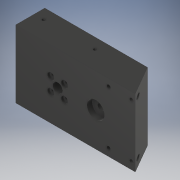
# Autodesk Inventor part: BA03
Saved by Autodesk Inventor 2017 (Build 210142000, 142)
## iProperties
Created: 2018-10-18
Part Number: BA03
Material: ABS Plastic
Document SubType Name: Modeling
Designer: Administrator
Density: 1.06 g/cm^3
Appearance: Smooth - Black
Author: Administrator
Autodesk Inventor part; units mm, degrees
ref_plane "YZ Plane" through (0, 0, 0) normal (1, 0, 0) x (0, 1, 0)
ref_plane "XZ Plane" through (0, 0, 0) normal (0, 1, 0) x (-1, 0, 0)
ref_plane "XY Plane" through (0, 0, 0) normal (0, 0, 1) x (1, 0, 0)
sketch "Sketch1" plane through (0, 0, 0) normal (0, 0, 1) x (1, 0, 0)
  line L0 (0, 0) -> (110, 0)
  line L1 (110, 0) -> (110, 75)
  line L2 (110, 75) -> (0, 75)
  line L3 (0, 75) -> (0, 0)
  circle A0 centre (80, 30.55) radius 4.5
  circle A1 centre (30, 30.55) radius 4
  line L4 (30, 30.55) -> (80, 30.55) construction
  dimension "d0" = 110
  dimension "d1" = 75
  dimension "d2" = 9
  dimension "d3" = 8
  dimension "d4" = 50
  dimension "d5" = 30
  dimension "d80" = 44.45
  constraints: 10 end point, 2 centre point, 2 horizontal, 2 parallel, 1 perpendicular
  measures "d0" distance of L2.end L1.end
  measures "d1" distance of L1.end L0.end
  measures "d2" diameter of A0
  measures "d3" diameter of A1
  measures "d4" distance of L4.start L4.end
  measures "d5" distance from line of L1 L4.end
  measures "d80" distance between parallel lines of L2 L4
extrude "Extrusion1" add sketch "Sketch1" along normal blind 10
sketch "Sketch2" plane through (0, 75, 0) normal (0, 1, 0) x (1, 0, 0)
  line L0 (110, -10) -> (0, -10) projected
  line L1 (0, -10) -> (110, -10)
  line L2 (110, -10) -> (110, 28.1)
  line L3 (110, 28.1) -> (0, 28.1)
  line L4 (0, 28.1) -> (0, -10)
  point P0 (0, 0)
  dimension "d8" = 38.1
  constraints: 8 end point, 2 parallel, 1 horizontal, 1 perpendicular
  measures "d8" distance of L3.end L0.end
extrude "Extrusion2" add sketch "Sketch2" against normal blind 10
sketch "Sketch3" plane through (110, 0, 10) normal (1, 0, 0) x (0, 0, -1)
  line L0 (38.1, 65) -> (10, 65) projected
  line L1 (10, 0) -> (10, 65) projected
  line L2 (10, 0) -> (38.1, 65)
  constraints: 2 end point
extrude "Extrusion3" add sketch "Sketch3" against normal blind 10
sketch "Sketch4" plane through (0, 0, 10) normal (-1, 0, 0) x (0, 0, 1)
  line L0 (-10, 65) -> (-10, 0) projected
  line L1 (-38.1, 65) -> (-10, 65) projected
  line L2 (-38.1, 65) -> (-10, 0) projected
  point P0 (-10, 0)
extrude "Extrusion4" add sketch "Sketch4" against normal blind 10
sketch "Sketch6" plane through (0, 65, 0) normal (0, -1, 0) x (1, 0, 0)
  line L0 (110, -28.1) -> (110, 10) projected
  line L1 (110, 0) -> (135, 0)
  line L2 (135, 0) -> (135, -28.1)
  line L3 (135, -28.1) -> (110, -28.1)
  line L4 (110, -28.1) -> (110, 0)
  line L5 (0, 0) -> (-25, 0)
  line L6 (-25, 0) -> (-25, -28.1)
  line L7 (-25, -28.1) -> (0, -28.1)
  line L8 (0, -28.1) -> (0, 0)
  line L9 (10, -28.1) -> (100, -28.1) projected
  circle A0 centre (122.5, -14.05) radius 2
  circle A1 centre (-12.5, -14.05) radius 2
  point P0 (135, -14.05)
  point P1 (-25, -14.05)
  point P2 (-12.5, -28.1)
  point P3 (122.5, -28.1)
  dimension "d17" = 25
  dimension "d18" = 25
  dimension "d19" = 4
  dimension "d20" = 4
  constraints: 16 end point, 4 horizontal alignment, 4 midpoint, 4 parallel, 2 centre point, 2 horizontal, 2 perpendicular, 2 vertical alignment, 1 coincident, 1 point on line
  measures "d17" distance of L6.end L7.end
  measures "d18" distance of L2.end L3.end
  measures "d19" diameter of A0
  measures "d20" diameter of A1
extrude "Extrusion5" add sketch "Sketch6" against normal blind 10
sketch "Sketch7" plane through (0, 65, 0) normal (0, -1, 0) x (1, 0, 0)
  line L0 (110, 0) -> (135, 0) projected
  line L1 (110, 0) -> (135, 0)
  line L2 (135, 0) -> (135, 10)
  line L3 (135, 10) -> (110, 10)
  line L4 (110, 10) -> (110, 0)
  line L5 (0, 0) -> (10, 0) projected
  line L6 (0, 0) -> (-25, 0)
  line L7 (-25, 0) -> (-25, 10)
  line L8 (-25, 10) -> (0, 10)
  line L9 (0, 10) -> (0, 0)
  point P0 (0, 10)
  point P1 (-25, 0)
  constraints: 16 end point, 4 parallel, 2 horizontal, 2 horizontal alignment, 2 perpendicular, 2 vertical alignment
extrude "Extrusion6" add sketch "Sketch7" against normal blind 10
sketch "Sketch8" plane through (0, 65, 0) normal (0, -1, 0) x (1, 0, 0)
  circle A0 centre (122.5, -14.05) radius 2 projected
  line L0 (10, -28.1) -> (100, -28.1) projected
  circle A1 centre (55, -14.05) radius 2
  point P0 (0, 0)
  point P1 (55, -28.1)
  dimension "d25" = 4
  constraints: 1 centre point, 1 horizontal alignment, 1 midpoint, 1 vertical alignment
  measures "d25" diameter of A1
extrude "Extrusion7" cut sketch "Sketch8" against normal through all contours A1
sketch "Sketch11" plane through (0, 0, 10) normal (0, 0, 1) x (1, 0, 0)
  line L0 (30, 23.55) -> (45.5, 23.55) construction
  circle A0 centre (30, 30.55) radius 4 construction
  circle A1 centre (45.5, 23.55) radius 1.5
  line L1 (30, 23.55) -> (37.75, 36.9734) construction
  circle A2 centre (37.75, 36.9734) radius 1.5
  line L2 (30, 23.55) -> (22.25, 36.9734) construction
  circle A3 centre (22.25, 36.9734) radius 1.5
  line L3 (30, 23.55) -> (14.5, 23.55) construction
  circle A4 centre (14.5, 23.55) radius 1.5
  line L4 (30, 23.55) -> (22.25, 10.1266) construction
  circle A5 centre (22.25, 10.1266) radius 1.5
  line L5 (30, 23.55) -> (37.75, 10.1266) construction
  circle A6 centre (37.75, 10.1266) radius 1.5
  point P0 (0, 0)
  dimension "d31" = 15.5
  dimension "d32" = 7
  dimension "d33" = 3
  dimension "d36" = 360
  constraints: 12 end point, 8 coincident, 6 centre point, 1 horizontal, 1 vertical alignment, 29 other
  measures "d31" distance of L0.start L0.end
  measures "d32" distance of L0.start A0.centre
  measures "d33" diameter of A1
extrude "Extrusion9" cut sketch "Sketch11" against normal through all
sketch "Sketch12" plane through (0, 0, 0) normal (0, 0, -1) x (-1, 0, 0)
  circle A0 centre (-30, 30.55) radius 4 projected
  circle A1 centre (-30, 30.55) radius 6.5
  point P0 (0, 0)
  dimension "d40" = 13
  constraints: 1 centre point, 1 coincident
  measures "d40" diameter of A1
extrude "Extrusion10" cut sketch "Sketch12" against normal through all
sketch "Sketch13" plane through (0, 0, 10) normal (0, 0, 1) x (1, 0, 0)
  circle A0 centre (45.5, 23.55) radius 1.5 projected
  circle A1 centre (14.5, 23.55) radius 1.5 projected
  circle A2 centre (22.25, 36.9734) radius 1.5 projected
  circle A3 centre (37.75, 36.9734) radius 1.5 projected
  circle A4 centre (37.75, 10.1266) radius 1.5 projected
  circle A5 centre (22.25, 10.1266) radius 1.5 projected
  circle A6 centre (14.5, 23.55) radius 4
  circle A7 centre (22.25, 36.9734) radius 4
  circle A8 centre (37.75, 36.9734) radius 4
  circle A9 centre (45.5, 23.55) radius 4
  circle A10 centre (37.75, 10.1266) radius 4
  circle A11 centre (22.25, 10.1266) radius 4
  point P0 (0, 0)
  dimension "d43" = 8
  dimension "d44" = 8
  dimension "d45" = 8
  dimension "d46" = 8
  dimension "d47" = 8
  dimension "d48" = 8
  constraints: 6 centre point, 6 coincident
  measures "d43" diameter of A6
  measures "d44" diameter of A7
  measures "d45" diameter of A8
  measures "d46" diameter of A9
  measures "d47" diameter of A10
  measures "d48" diameter of A11
extrude "Extrusion11" cut sketch "Sketch13" against normal blind 3 contours A0 | A1 | A2 | A3 | A4 | A5 | A6 | A7 | A8 | A9 | A10 | A11
sketch "Sketch15" plane through (0, 0, 10) normal (0, 0, 1) x (1, 0, 0)
  line L0 (135, 75) -> (-25, 75) projected
  line L1 (110, 75) -> (0, 75)
  line L2 (0, 75) -> (0, -13.9)
  line L3 (0, -13.9) -> (110, -13.9)
  line L4 (110, -13.9) -> (110, 75)
  line L5 (100, 0) -> (110, 0) projected
  line L6 (110, 0) -> (0, 0)
  line L7 (0, 0) -> (0, -13.9)
  line L8 (0, -13.9) -> (110, -13.9)
  line L9 (110, -13.9) -> (110, 0)
  dimension "d54" = 88.9
  constraints: 16 end point, 4 parallel, 2 horizontal, 2 perpendicular, 2 vertical alignment, 1 point on line
  measures "d54" distance between parallel lines of L0 L3
extrude "Extrusion13" add sketch "Sketch15" against normal blind 10 contours L4 L3 L2 L6 L5
sketch "Sketch16" plane through (0, -13.9, 10) normal (0, -1, 0) x (1, 0, 0)
  line L0 (0, 0) -> (0, -38.1) projected
  line L1 (10, -10) -> (10, -38.1) projected
  line L2 (0, 0) -> (10, 0)
  line L3 (10, 0) -> (10, -38.1)
  line L4 (10, -38.1) -> (0, -38.1)
  line L5 (0, -38.1) -> (0, 0)
  line L6 (135, 0) -> (110, 0) projected
  line L7 (100, -38.1) -> (100, -10) projected
  line L8 (110, 0) -> (100, 0)
  line L9 (100, 0) -> (100, -38.1)
  line L10 (100, -38.1) -> (110, -38.1)
  line L11 (110, -38.1) -> (110, 0)
  point P0 (0, -10)
  constraints: 16 end point, 4 parallel, 2 horizontal, 2 perpendicular
extrude "Extrusion14" add sketch "Sketch16" against normal blind 88.9
sketch "Sketch17" plane through (100, -13.9, -28.1) normal (0, -1, 0) x (1, 0, 0)
  line L0 (10, 0) -> (10, 38.1) projected
  line L1 (10, 0) -> (-100, 0)
  line L2 (-100, 0) -> (-100, 38.1)
  line L3 (-100, 38.1) -> (10, 38.1)
  line L4 (10, 38.1) -> (10, 0)
  point P0 (-100, 28.1)
  constraints: 8 end point, 2 parallel, 1 coincident, 1 horizontal, 1 perpendicular
extrude "Extrusion15" add sketch "Sketch17" against normal blind 10
sketch "Sketch18" plane through (0, -13.9, 10) normal (0, -1, 0) x (1, 0, 0)
  line L0 (0, -38.1) -> (110, -38.1) projected
  line L1 (110, 0) -> (110, -38.1) projected
  line L2 (0, 0) -> (110, 0) projected
  line L3 (0, 0) -> (0, -38.1) projected
  circle A0 centre (122.5, -24.05) radius 2 projected
  line L4 (110, -38.1) -> (110, 0) projected
  line L5 (135, -38.1) -> (110, -38.1) projected
  line L6 (135, -38.1) -> (135, 0) projected
  line L7 (135, 0) -> (110, 0) projected
  circle A1 centre (-12.5, -24.05) radius 2 projected
  line L8 (-25, 0) -> (-25, -38.1) projected
  line L9 (-25, -38.1) -> (0, -38.1) projected
  line L10 (0, 0) -> (0, -38.1) projected
  line L11 (-25, 0) -> (0, 0) projected
  point P0 (0, -10)
extrude "Extrusion16" add sketch "Sketch18" against normal blind 10 contours L9 L8 L11 L3 | L1 L7 L6 L5
sketch "Sketch19" plane through (135, -13.9, -28.1) normal (0, -1, 0) x (1, 0, 0)
  circle A0 centre (-80, 14.05) radius 2 projected
  circle A1 centre (-80, 14.05) radius 2 projected
  point P0 (-135, 28.1)
extrude "Extrusion17" cut sketch "Sketch19" against normal blind 10
sketch "Sketch20" plane through (0, 0, 10) normal (0, 0, 1) x (1, 0, 0)
  line L0 (135, 65) -> (110, 65) projected
  line L1 (110, -3.9) -> (110, 65) projected
  line L2 (135, 65) -> (110, 65)
  line L3 (110, 65) -> (110, -3.9)
  line L4 (110, -3.9) -> (135, -3.9)
  line L5 (135, -3.9) -> (135, 65)
  line L6 (0, -3.9) -> (-25, -3.9) projected
  line L7 (-25, 65) -> (0, 65) projected
  line L8 (0, -3.9) -> (-25, -3.9)
  line L9 (-25, -3.9) -> (-25, 65)
  line L10 (-25, 65) -> (0, 65)
  line L11 (0, 65) -> (0, -3.9)
  point P0 (0, 0)
  constraints: 16 end point, 4 parallel, 2 horizontal, 2 perpendicular
extrude "Extrusion18" add sketch "Sketch20" against normal blind 10
sketch "Sketch21" plane through (0, 0, 0) normal (0, 0, -1) x (-1, 0, 0)
  circle A0 centre (-80, 30.55) radius 4.5 projected
  circle A1 centre (-80, 30.55) radius 22.5
  point P0 (0, 0)
  dimension "d67" = 45
  constraints: 1 centre point, 1 coincident
  measures "d67" diameter of A1
extrude "Extrusion19" add sketch "Sketch21" along normal blind 28.1
sketch "Sketch22" plane through (80, 30.55, -28.1) normal (0, 0, -1) x (0, 1, 0)
  circle A0 centre (0, 0) radius 4.5 projected
  circle A1 centre (0, 0) radius 4.5 projected
  circle A2 centre (0, 0) radius 11.5
  point P0 (-30.55, -80)
  dimension "d70" = 23
  constraints: 1 centre point, 1 coincident
  measures "d70" diameter of A2
extrude "Extrusion20" cut sketch "Sketch22" against normal blind 7
sketch "Sketch23" plane through (0, 0, 10) normal (0, 0, 1) x (1, 0, 0)
  circle A0 centre (80, 30.55) radius 4.5 projected
  circle A1 centre (80, 30.55) radius 11.5
  point P0 (0, 0)
  dimension "d73" = 23
  constraints: 1 centre point, 1 coincident
  measures "d73" diameter of A1
extrude "Extrusion21" cut sketch "Sketch23" against normal blind 7
sketch "Sketch24" plane through (-25, 75, -28.1) normal (0, 1, 0) x (1, 0, 0)
  line L0 (160, 0) -> (160, -28.1) projected
  line L1 (160, 0) -> (160, -38.1) projected
  line L2 (0, -38.1) -> (160, -38.1) projected
  line L3 (160, -38.1) -> (181.997, -38.1)
  line L4 (160, 0) -> (0, 0) projected
  line L5 (181.997, -38.1) -> (160, 0)
  point P0 (25, -28.1)
  dimension "d79" = 30
  constraints: 4 end point, 1 horizontal
  measures "d79" angle of L0 L5
extrude "Extrusion22" add sketch "Sketch24" against normal blind 88.9
sketch "Sketch25" plane through (-25, -13.9, -28.1) normal (0, -1, 0) x (1, 0, 0)
  line L0 (135, 28.1) -> (135, 0) projected
  line L1 (135, 0) -> (135, 28.1) projected
  line L2 (135, 28.1) -> (135, 0) projected
  line L3 (135, 0) -> (135, 38.1)
  line L4 (0, 38.1) -> (181.997, 38.1) projected
  line L5 (160, 0) -> (181.997, 38.1) projected
  line L6 (135, 0) -> (156.997, 38.1)
  line L7 (135, 38.1) -> (156.997, 38.1)
  line L8 (160, 0) -> (135, 0) projected
  line L9 (160, 0) -> (135, 0)
  line L10 (135, 0) -> (156.997, 38.1)
  line L11 (181.997, 38.1) -> (160, 0)
  line L12 (181.997, 38.1) -> (156.997, 38.1)
  point P0 (25, 28.1)
  constraints: 14 end point, 3 collinear, 2 parallel, 2 point on line, 1 vertical
extrude "Extrusion23" cut sketch "Sketch25" against normal through all contours L6 L4 L5 L8
sketch "Sketch26" plane through (0, 65, 0) normal (0, -1, 0) x (1, 0, 0)
  line L0 (110, -28.1) -> (126.2235, 0) projected
  line L1 (126.2235, 0) -> (110, 0) projected
  line L2 (110, -28.1) -> (110, 0) projected
  point P0 (0, 0)
extrude "Extrusion24" add sketch "Sketch26" along normal blind 70
sketch "Sketch28" plane through (0, 0, 10) normal (0, 0, 1) x (1, 0, 0)
  circle A0 centre (80, 30.55) radius 4.5 construction
  circle A1 centre (80, 30.55) radius 4.5 construction
  line L0 (80, 30.55) -> (131.997, 30.55) construction
  line L1 (131.997, -13.9) -> (131.997, 75) projected
  line L2 (126.997, 65.55) -> (96.997, 65.55) construction
  circle A2 centre (96.997, 65.55) radius 2.5
  circle A3 centre (126.997, 65.55) radius 2.5
  point P0 (0, 0)
  point P1 (111.997, 65.55)
  point P2 (111.997, 65.55)
  dimension "d96" = 30
  dimension "d98" = 5
  dimension "d99" = 5
  dimension "d106" = 35
  dimension "d107" = 20
  constraints: 4 end point, 3 coincident, 2 centre point, 2 midpoint, 1 horizontal
  measures "d96" distance of L2.start L2.end
  measures "d98" diameter of A2
  measures "d99" diameter of A3
  measures "d106" distance from line of L0 point (111.997, 65.55)
  measures "d107" distance from line of L1 point (111.997, 65.55)
extrude "Extrusion26" cut sketch "Sketch28" against normal through all
ref_plane "Work Plane1" through (-25, 30.55, 10) normal (0, 1, 0) x (1, 0, 0)
mirror "Mirror1" about plane through (-25, 30.55, 10) normal (0, 1, 0) of "Extrusion26"
sketch "Sketch30" plane through (37.75, 10.1266, 7) normal (0, 0, 1) x (1, 0, 0)
  arc A0 (-1.9476, 23.353) -> (-3.7946, 25.5813) centre (-7.75, 20.4234) ccw projected
  arc A1 (-1.9476, 23.353) -> (-3.7946, 25.5813) centre (0, 26.8468) ccw projected
  circle A2 centre (0, 26.8468) radius 1.5 projected
  circle A3 centre (7.75, 13.4234) radius 1.5 projected
  circle A4 centre (7.75, 13.4234) radius 4 projected
  circle A5 centre (0, 0) radius 1.5 projected
  circle A6 centre (0, 0) radius 4 projected
  circle A7 centre (-15.5, 0) radius 1.5 projected
  circle A8 centre (-15.5, 0) radius 4 projected
  circle A9 centre (-23.25, 13.4234) radius 1.5 projected
  circle A10 centre (-23.25, 13.4234) radius 4 projected
  arc A11 (-11.7054, 25.5813) -> (-13.5524, 23.353) centre (-7.75, 20.4234) ccw projected
  arc A12 (-11.7054, 25.5813) -> (-13.5524, 23.353) centre (-15.5, 26.8468) ccw projected
  circle A13 centre (-15.5, 26.8468) radius 1.5 projected
  point P0 (-37.75, -10.1266)
extrude "Extrusion27" add sketch "Sketch30" along normal blind 3 and the other way blind 7 contours A0 A1 | A2 | A3 | A4 | A5 | A6 | A7 | A8 | A9 | A10 | A11 A12 | A13
sketch "Sketch31" plane through (0, 0, 0) normal (0, 0, -1) x (-1, 0, 0)
  circle A0 centre (-30, 30.55) radius 6.5 projected
  circle A1 centre (-21, 21.55) radius 2
  line L0 (-30, 30.55) -> (-21, 21.55) construction
  line L1 (-30, 30.55) -> (-20.5857, 30.55) construction
  line L2 (-30, 30.55) -> (-30, 39.9643) construction
  line L3 (-30, 30.55) -> (-21, 39.55) construction
  circle A2 centre (-21, 39.55) radius 2
  line L4 (-30, 30.55) -> (-39.4143, 30.55) construction
  line L5 (-30, 30.55) -> (-39, 39.55) construction
  circle A3 centre (-39, 39.55) radius 2
  line L6 (-30, 30.55) -> (-30, 21.1357) construction
  line L7 (-30, 30.55) -> (-39, 21.55) construction
  circle A4 centre (-39, 21.55) radius 2
  point P0 (0, 0)
  dimension "d112" = 4
  dimension "d113" = 12.7279
  dimension "d114" = 45
  dimension "d117" = 360
  constraints: 16 end point, 4 centre point, 2 coincident, 1 horizontal, 23 other
  measures "d112" diameter of A1
  measures "d113" distance of L0.end L0.start
  measures "d114" angle of L1 L0
extrude "Extrusion28" cut sketch "Sketch31" against normal through all contours A1 | A2 | A3 | A4
sketch "Sketch32" plane through (0, 0, 10) normal (0, 0, 1) x (1, 0, 0)
  circle A0 centre (21, 21.55) radius 2 projected
  circle A1 centre (30, 30.55) radius 6.5 construction
  circle A2 centre (21, 21.55) radius 4.5
  circle A3 centre (39, 21.55) radius 4.5
  circle A4 centre (39, 39.55) radius 4.5
  circle A5 centre (21, 39.55) radius 4.5
  point P0 (0, 0)
  dimension "d121" = 9
  dimension "d124" = 360
  constraints: 4 centre point, 1 coincident, 9 other
  measures "d121" diameter of A2
extrude "Extrusion29" cut sketch "Sketch32" against normal blind 3 contours A0 | A2 | A3 | A4 | A5
body "Solid1"
